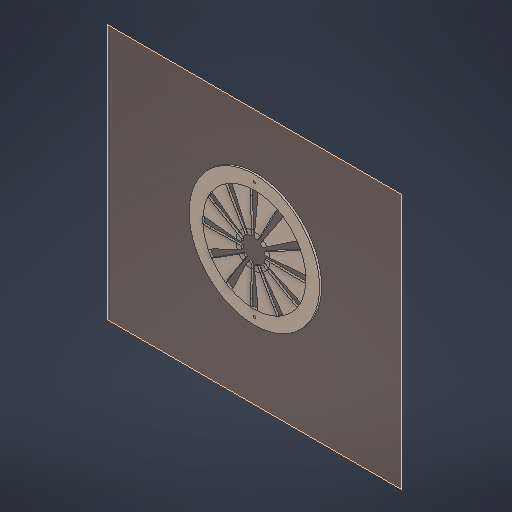
# Autodesk Inventor part: Prressure plate
Saved by Autodesk Inventor 2026.3 (Build 303398000, 398)
## iProperties
Created: 2026-07-26
Part Number: Prressure plate
Material: Generic
Document SubType Name: Sheet Metal
Designer: matot
Density: 1 g/cm^3
Sheet Metal Rule: Default_mm
Appearance: Default
Author: matot
Autodesk Inventor part; units mm, degrees
ref_plane "YZ Plane" through (0, 0, 0) normal (1, 0, 0) x (0, 1, 0)
ref_plane "XZ Plane" through (0, 0, 0) normal (0, 1, 0) x (-1, 0, 0)
ref_plane "XY Plane" through (0, 0, 0) normal (0, 0, 1) x (1, 0, 0)
sketch "Sketch1" plane through (0, 0, 0) normal (1, 0, 0) x (0, 1, 0)
  line L0 (0, 0) -> (95, 0)
  line L1 (95, 0) -> (95, 3)
  line L2 (0, 3) -> (0, 0)
  line L3 (0, 0) -> (38.25, 0)
  line L4 (25, 5) -> (0, 5)
  line L5 (0, 5) -> (0, 0)
  line L6 (0, 5) -> (25, 5)
  line L7 (25, 3) -> (25, 2)
  line L8 (25, 2) -> (0, 2)
  line L9 (0, 2) -> (0, 5)
  line L10 (95, 3) -> (75, 3)
  line L11 (75, 0) -> (95, 0)
  line L12 (95, 0) -> (95, 3)
  line L13 (75, 0) -> (25, 2)
  line L14 (75, 3) -> (25, 5)
  point P0 (0, 3.5)
  point P1 (25, 3.5)
  point P2 (0, 2)
  point P3 (95, 1.5)
  dimension "d2" = 5
  dimension "d3" = 25
  dimension "d4" = 3
  dimension "d5" = 3
  dimension "d6" = 25
  dimension "d52" = 50
  dimension "d53" = 50
  dimension "d54" = 20
  constraints: 30 end point, 5 parallel, 4 horizontal, 3 point on line, 2 midpoint, 2 perpendicular
  measures "d2" distance of L0.start L4.end
  measures "d3" distance of L4.start L4.end
  measures "d4" distance of L6.end L7.end
  measures "d5" distance of L0.end L1.end
  measures "d6" distance of point (0, 3.5) point (25, 3.5)
  measures "d52" horizontal distance of L11.start L7.end
  measures "d53" horizontal distance of L4.start L10.end
  measures "d54" horizontal distance of L10.end point (95, 1.5)
revolve "Revolution1" add sketch "Sketch1" angle 360 about axis through (0, 0, 5) along (0, 0, -1) contours L2 L5 L4 L14 L10 L1 L0 L13 L8
sketch "Sketch2" plane through (0, 0, 5) normal (0, 0, 1) x (1, 0, 0)
  circle A0 centre (0, 0) radius 17.5
  dimension "d9" = 35
  constraints: 1 centre point, 1 coincident
  measures "d9" diameter of A0
extrude "Extrusion1" cut sketch "Sketch2" against normal through all
ref_plane "Work Plane1" through (0, 0, 5) normal (0, 0, 1) x (1, 0, 0)
sketch "Sketch6" plane through (0, 0, 3) normal (0, 0, 1) x (1, 0, 0)
  point P0 (0, 0)
  point P1 (0, 85)
  point P2 (0, -85)
  dimension "d86" = 85
  dimension "d87" = 85
  measures "d86" distance of point (0, 0) point (0, -85)
  measures "d87" distance of point (0, 0) point (0, 85)
hole "Hole1" at (0, 85, 3) at (0, -85, 3) direction (0, 0, -1) diameter 3.4587 end through all thread size "M4x0.5" class "6H" standard "ISO Metric profile"
sketch "Sketch7" plane through (0, 0, 5) normal (0, 0, 1) x (1, 0, 0)
  circle A0 centre (0, 0) radius 25 projected
  line L0 (-5, 75) -> (5, 75)
  line L1 (5, 75) -> (5, 65)
  line L2 (-5, 65) -> (-5, 75)
  circle A1 centre (0, 0) radius 17.5 projected
  line L3 (2.5, 24.8747) -> (2.5, 17.3205)
  line L4 (2.5, 17.3205) -> (-2.5, 17.3205)
  line L5 (-2.5, 17.3205) -> (-2.5, 24.8747)
  line L6 (5, 65) -> (2.5, 24.8747)
  line L7 (-5, 65) -> (-2.5, 24.8747)
  line L8 (5, 65) -> (2.5, 65)
  line L9 (-41.8301, 62.4519) -> (-33.1699, 67.4519)
  line L10 (-36.8301, 53.7917) -> (-41.8301, 62.4519)
  line L11 (-36.8301, 53.7917) -> (-14.6024, 20.2921)
  line L12 (-10.8253, 13.75) -> (-14.6024, 20.2921)
  line L13 (-6.4952, 16.25) -> (-10.8253, 13.75)
  line L14 (-10.2723, 22.7921) -> (-6.4952, 16.25)
  line L15 (-28.1699, 58.7917) -> (-10.2723, 22.7921)
  line L16 (-33.1699, 67.4519) -> (-28.1699, 58.7917)
  line L17 (-67.4519, 33.1699) -> (-62.4519, 41.8301)
  line L18 (-58.7917, 28.1699) -> (-67.4519, 33.1699)
  line L19 (-58.7917, 28.1699) -> (-22.7921, 10.2723)
  line L20 (-16.25, 6.4952) -> (-22.7921, 10.2723)
  line L21 (-13.75, 10.8253) -> (-16.25, 6.4952)
  line L22 (-20.2921, 14.6024) -> (-13.75, 10.8253)
  line L23 (-53.7917, 36.8301) -> (-20.2921, 14.6024)
  line L24 (-62.4519, 41.8301) -> (-53.7917, 36.8301)
  line L25 (-75, -5) -> (-75, 5)
  line L26 (-65, -5) -> (-75, -5)
  line L27 (-65, -5) -> (-24.8747, -2.5)
  line L28 (-17.3205, -2.5) -> (-24.8747, -2.5)
  line L29 (-17.3205, 2.5) -> (-17.3205, -2.5)
  line L30 (-24.8747, 2.5) -> (-17.3205, 2.5)
  line L31 (-65, 5) -> (-24.8747, 2.5)
  line L32 (-75, 5) -> (-65, 5)
  line L33 (-62.4519, -41.8301) -> (-67.4519, -33.1699)
  line L34 (-53.7917, -36.8301) -> (-62.4519, -41.8301)
  line L35 (-53.7917, -36.8301) -> (-20.2921, -14.6024)
  line L36 (-13.75, -10.8253) -> (-20.2921, -14.6024)
  line L37 (-16.25, -6.4952) -> (-13.75, -10.8253)
  line L38 (-22.7921, -10.2723) -> (-16.25, -6.4952)
  line L39 (-58.7917, -28.1699) -> (-22.7921, -10.2723)
  line L40 (-67.4519, -33.1699) -> (-58.7917, -28.1699)
  line L41 (-33.1699, -67.4519) -> (-41.8301, -62.4519)
  line L42 (-28.1699, -58.7917) -> (-33.1699, -67.4519)
  line L43 (-28.1699, -58.7917) -> (-10.2723, -22.7921)
  line L44 (-6.4952, -16.25) -> (-10.2723, -22.7921)
  line L45 (-10.8253, -13.75) -> (-6.4952, -16.25)
  line L46 (-14.6024, -20.2921) -> (-10.8253, -13.75)
  line L47 (-36.8301, -53.7917) -> (-14.6024, -20.2921)
  line L48 (-41.8301, -62.4519) -> (-36.8301, -53.7917)
  line L49 (5, -75) -> (-5, -75)
  line L50 (5, -65) -> (5, -75)
  line L51 (5, -65) -> (2.5, -24.8747)
  line L52 (2.5, -17.3205) -> (2.5, -24.8747)
  line L53 (-2.5, -17.3205) -> (2.5, -17.3205)
  line L54 (-2.5, -24.8747) -> (-2.5, -17.3205)
  line L55 (-5, -65) -> (-2.5, -24.8747)
  line L56 (-5, -75) -> (-5, -65)
  line L57 (41.8301, -62.4519) -> (33.1699, -67.4519)
  line L58 (36.8301, -53.7917) -> (41.8301, -62.4519)
  line L59 (36.8301, -53.7917) -> (14.6024, -20.2921)
  line L60 (10.8253, -13.75) -> (14.6024, -20.2921)
  line L61 (6.4952, -16.25) -> (10.8253, -13.75)
  line L62 (10.2723, -22.7921) -> (6.4952, -16.25)
  line L63 (28.1699, -58.7917) -> (10.2723, -22.7921)
  line L64 (33.1699, -67.4519) -> (28.1699, -58.7917)
  line L65 (67.4519, -33.1699) -> (62.4519, -41.8301)
  line L66 (58.7917, -28.1699) -> (67.4519, -33.1699)
  line L67 (58.7917, -28.1699) -> (22.7921, -10.2723)
  line L68 (16.25, -6.4952) -> (22.7921, -10.2723)
  line L69 (13.75, -10.8253) -> (16.25, -6.4952)
  line L70 (20.2921, -14.6024) -> (13.75, -10.8253)
  line L71 (53.7917, -36.8301) -> (20.2921, -14.6024)
  line L72 (62.4519, -41.8301) -> (53.7917, -36.8301)
  line L73 (75, 5) -> (75, -5)
  line L74 (65, 5) -> (75, 5)
  line L75 (65, 5) -> (24.8747, 2.5)
  line L76 (17.3205, 2.5) -> (24.8747, 2.5)
  line L77 (17.3205, -2.5) -> (17.3205, 2.5)
  line L78 (24.8747, -2.5) -> (17.3205, -2.5)
  line L79 (65, -5) -> (24.8747, -2.5)
  line L80 (75, -5) -> (65, -5)
  line L81 (62.4519, 41.8301) -> (67.4519, 33.1699)
  line L82 (53.7917, 36.8301) -> (62.4519, 41.8301)
  line L83 (53.7917, 36.8301) -> (20.2921, 14.6024)
  line L84 (13.75, 10.8253) -> (20.2921, 14.6024)
  line L85 (16.25, 6.4952) -> (13.75, 10.8253)
  line L86 (22.7921, 10.2723) -> (16.25, 6.4952)
  line L87 (58.7917, 28.1699) -> (22.7921, 10.2723)
  line L88 (67.4519, 33.1699) -> (58.7917, 28.1699)
  line L89 (33.1699, 67.4519) -> (41.8301, 62.4519)
  line L90 (28.1699, 58.7917) -> (33.1699, 67.4519)
  line L91 (28.1699, 58.7917) -> (10.2723, 22.7921)
  line L92 (6.4952, 16.25) -> (10.2723, 22.7921)
  line L93 (10.8253, 13.75) -> (6.4952, 16.25)
  line L94 (14.6024, 20.2921) -> (10.8253, 13.75)
  line L95 (36.8301, 53.7917) -> (14.6024, 20.2921)
  line L96 (41.8301, 62.4519) -> (36.8301, 53.7917)
  point P0 (0, 25)
  point P1 (0, 75)
  point P2 (-37.5, 64.9519)
  point P3 (-12.5, 21.6506)
  point P4 (-64.9519, 37.5)
  point P5 (-21.6506, 12.5)
  point P6 (-75, 0)
  point P7 (-25, 0)
  point P8 (-64.9519, -37.5)
  point P9 (-21.6506, -12.5)
  point P10 (-37.5, -64.9519)
  point P11 (-12.5, -21.6506)
  point P12 (0, -75)
  point P13 (0, -25)
  point P14 (37.5, -64.9519)
  point P15 (12.5, -21.6506)
  point P16 (64.9519, -37.5)
  point P17 (21.6506, -12.5)
  point P18 (75, 0)
  point P19 (25, 0)
  point P20 (64.9519, 37.5)
  point P21 (21.6506, 12.5)
  point P22 (37.5, 64.9519)
  point P23 (12.5, 21.6506)
  point P24 (0, 17.3205)
  point P25 (0, 65)
  point P26 (-8.6603, 15)
  point P27 (-30.3349, 57.5417)
  point P28 (-15, 8.6603)
  point P29 (-55.0417, 34.6651)
  point P30 (-17.3205, 0)
  point P31 (-65, 2.5)
  point P32 (-15, -8.6603)
  point P33 (-57.5417, -30.3349)
  point P34 (-8.6603, -15)
  point P35 (-34.6651, -55.0417)
  point P36 (0, -17.3205)
  point P37 (-2.5, -65)
  point P38 (8.6603, -15)
  point P39 (30.3349, -57.5417)
  point P40 (15, -8.6603)
  point P41 (55.0417, -34.6651)
  point P42 (17.3205, 0)
  point P43 (65, -2.5)
  point P44 (15, 8.6603)
  point P45 (57.5417, 30.3349)
  point P46 (8.6603, 15)
  point P47 (34.6651, 55.0417)
  dimension "d97" = 360
  dimension "d99" = 5
  dimension "d100" = 0
  dimension "d101" = 0
  dimension "d102" = 10
  dimension "d103" = 0
  dimension "d104" = 10
  dimension "d107" = 360
  constraints: 194 end point, 12 point on line, 3 parallel, 2 point on circle, 1 horizontal, 1 midpoint, 1 perpendicular, 244 other
  measures "d99" distance of L3.end L4.end
  measures "d100" horizontal distance of point (0, 17.321) A0.start
  measures "d101" horizontal distance of point (0, 0) A0.start
  measures "d102" distance of L0.start L0.end
  measures "d103" horizontal distance of point (0, 65) point (0, 75)
  measures "d104" distance of L0.end L1.end
extrude "Extrusion5" cut sketch "Sketch7" against normal through all contours A0 L78 A1 L76 | A0 L75 L74 L73 L80 L79 | L86 A1 L84 A0 | A0 L83 L82 L81 L88 L87 | A1 L77 | L67 L66 L65 L72 L71 A0 | A0 L70 A1 L68 | L85 A1 | A1 L69 | L94 A1 L92 A0 | A0 L91 L90 L89 L96 L95 | L59 L58 L57 L64 L63 A0 | A0 L62 A1 L60 | L93 A1 | A1 L61 | L3 A1 L5 A0 | A0 L7 L2 L0 L1 L6 | L51 L50 L49 L56 L55 A0 | A0 L54 A1 L52 | L4 A1 | A1 L53 | L14 A1 L12 A0 | A0 L11 L10 L9 L16 L15 | L43 L42 L41 L48 L47 A0 | A0 L46 A1 L44 | L13 A1 | A1 L45 | L22 A1 L20 A0 | A0 L19 L18 L17 L24 L23 | L35 L34 L33 L40 L39 A0 | A0 L38 A1 L36 | L21 A1 | A1 L37 | L30 A1 L28 A0 | A0 L27 L26 L25 L32 L31 | L29 A1
equation "\"d93\" = Thickness"
equation "\"BendRadius\" = Thickness"
equation "\"BendReliefWidth\" = Thickness"
equation "\"BendReliefDepth\" = 0.5 * Thickness"
equation "\"CornerReliefSize\" = 4 * Thickness"
equation "\"MinimumRemnant\" = 2 * Thickness"
equation "\"TransitionRadius\" = BendRadius"
equation "\"JacobiRadiusSize\" = BendRadius"
equation "\"GapSize\" = Thickness"
equation "\"Thickness\" = 0.5"
body "Solid1"
